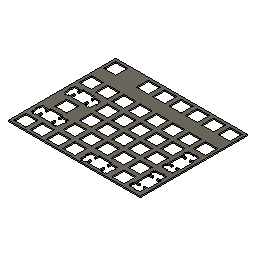
keeb plate v2 (Autodesk Fusion 360 design; units mm, degrees)
Autodesk Fusion 360 part; units mm, degrees
sketch "Sketch1" plane through (0, 0, 0) normal (0, 0, 1) x (1, 0, 0)
  line L0 (93.2552, -112.3061) -> (93.2552, -117.0063)
  line L1 (93.2552, -117.0063) -> (91.7301, -117.0063)
  line L2 (91.7301, -117.0063) -> (91.7301, -113.7761)
  line L3 (91.7301, -113.7761) -> (84.9798, -113.7761)
  line L4 (84.9798, -113.7761) -> (84.9798, -117.0063)
  line L5 (84.9798, -117.0063) -> (84.1548, -117.0063)
  line L6 (84.1548, -117.0063) -> (84.1548, -119.8064)
  line L7 (84.1548, -119.8064) -> (84.9798, -119.8064)
  line L8 (84.9798, -119.8064) -> (84.9798, -126.0767)
  line L9 (84.9798, -126.0767) -> (86.7049, -126.0767)
  line L10 (86.7049, -126.0767) -> (86.7049, -127.2767)
  line L11 (86.7049, -127.2767) -> (90.005, -127.2767)
  line L12 (90.005, -127.2767) -> (90.005, -126.0767)
  line L13 (90.005, -126.0767) -> (91.7301, -126.0767)
  line L14 (91.7301, -126.0767) -> (91.7301, -121.6065)
  line L15 (91.7301, -121.6065) -> (93.2552, -121.6065)
  line L16 (93.2552, -121.6065) -> (93.2552, -126.3067)
  line L17 (93.2552, -126.3067) -> (107.2558, -126.3067)
  line L18 (107.2558, -126.3067) -> (107.2558, -121.6065)
  line L19 (107.2558, -121.6065) -> (108.7809, -121.6065)
  line L20 (108.7809, -121.6065) -> (108.7809, -126.0767)
  line L21 (108.7809, -126.0767) -> (110.506, -126.0767)
  line L22 (110.506, -126.0767) -> (110.506, -127.2767)
  line L23 (110.506, -127.2767) -> (113.8061, -127.2767)
  line L24 (113.8061, -127.2767) -> (113.8061, -126.0767)
  line L25 (113.8061, -126.0767) -> (115.5312, -126.0767)
  line L26 (115.5312, -126.0767) -> (115.5312, -119.8064)
  line L27 (115.5312, -119.8064) -> (116.3562, -119.8064)
  line L28 (116.3562, -119.8064) -> (116.3562, -117.0063)
  line L29 (116.3562, -117.0063) -> (115.5312, -117.0063)
  line L30 (115.5312, -117.0063) -> (115.5312, -113.7761)
  line L31 (115.5312, -113.7761) -> (108.7809, -113.7761)
  line L32 (108.7809, -113.7761) -> (108.7809, -117.0063)
  line L33 (108.7809, -117.0063) -> (107.2558, -117.0063)
  line L34 (107.2558, -117.0063) -> (107.2558, -112.3061)
  line L35 (107.2558, -112.3061) -> (93.2552, -112.3061)
  line L36 (121.8305, -112.3061) -> (121.8305, -126.3067)
  line L37 (121.8305, -126.3067) -> (135.8321, -126.3067)
  line L38 (135.8321, -126.3067) -> (135.8321, -112.3061)
  line L39 (135.8321, -112.3061) -> (121.8305, -112.3061)
  line L40 (64.6789, -112.3061) -> (64.6789, -126.3067)
  line L41 (64.6789, -126.3067) -> (78.6795, -126.3067)
  line L42 (78.6795, -126.3067) -> (78.6795, -112.3061)
  line L43 (78.6795, -112.3061) -> (64.6789, -112.3061)
  line L44 (45.6281, -112.3061) -> (45.6281, -126.3067)
  line L45 (45.6281, -126.3067) -> (59.6287, -126.3067)
  line L46 (59.6287, -126.3067) -> (59.6287, -112.3061)
  line L47 (59.6287, -112.3061) -> (45.6281, -112.3061)
  line L48 (26.5772, -112.3061) -> (26.5772, -126.3067)
  line L49 (26.5772, -126.3067) -> (40.5778, -126.3067)
  line L50 (40.5778, -126.3067) -> (40.5778, -112.3061)
  line L51 (40.5778, -112.3061) -> (26.5772, -112.3061)
  line L52 (7.5263, -112.3061) -> (7.5263, -126.3067)
  line L53 (7.5263, -126.3067) -> (21.527, -126.3067)
  line L54 (21.527, -126.3067) -> (21.527, -112.3061)
  line L55 (21.527, -112.3061) -> (7.5263, -112.3061)
  line L56 (147.3826, -93.6802) -> (147.3826, -94.5053)
  line L57 (147.3826, -94.5053) -> (141.1123, -94.5053)
  line L58 (141.1123, -94.5053) -> (141.1123, -96.2303)
  line L59 (141.1123, -96.2303) -> (139.9123, -96.2303)
  line L60 (139.9123, -96.2303) -> (139.9123, -99.5305)
  line L61 (139.9123, -99.5305) -> (141.1123, -99.5305)
  line L62 (141.1123, -99.5305) -> (141.1123, -101.2556)
  line L63 (141.1123, -101.2556) -> (145.5826, -101.2556)
  line L64 (145.5826, -101.2556) -> (145.5826, -102.7806)
  line L65 (145.5826, -102.7806) -> (140.8823, -102.7806)
  line L66 (140.8823, -102.7806) -> (140.8823, -116.7813)
  line L67 (140.8823, -116.7813) -> (145.5826, -116.7813)
  line L68 (145.5826, -116.7813) -> (145.5826, -118.3063)
  line L69 (145.5826, -118.3063) -> (141.1123, -118.3063)
  line L70 (141.1123, -118.3063) -> (141.1123, -120.0314)
  line L71 (141.1123, -120.0314) -> (139.9123, -120.0314)
  line L72 (139.9123, -120.0314) -> (139.9123, -123.3315)
  line L73 (139.9123, -123.3315) -> (141.1123, -123.3315)
  line L74 (141.1123, -123.3315) -> (141.1123, -125.0566)
  line L75 (141.1123, -125.0566) -> (147.3826, -125.0566)
  line L76 (147.3826, -125.0566) -> (147.3826, -125.8817)
  line L77 (147.3826, -125.8817) -> (150.1828, -125.8817)
  line L78 (150.1828, -125.8817) -> (150.1828, -125.0566)
  line L79 (150.1828, -125.0566) -> (153.4129, -125.0566)
  line L80 (153.4129, -125.0566) -> (153.4129, -118.3063)
  line L81 (153.4129, -118.3063) -> (150.1828, -118.3063)
  line L82 (150.1828, -118.3063) -> (150.1828, -116.7813)
  line L83 (150.1828, -116.7813) -> (154.883, -116.7813)
  line L84 (154.883, -116.7813) -> (154.883, -102.7806)
  line L85 (154.883, -102.7806) -> (150.1828, -102.7806)
  line L86 (150.1828, -102.7806) -> (150.1828, -101.2556)
  line L87 (150.1828, -101.2556) -> (153.4129, -101.2556)
  line L88 (153.4129, -101.2556) -> (153.4129, -94.5053)
  line L89 (153.4129, -94.5053) -> (150.1828, -94.5053)
  line L90 (150.1828, -94.5053) -> (150.1828, -93.6802)
  line L91 (150.1828, -93.6802) -> (147.3826, -93.6802)
  line L92 (17.0518, -93.2552) -> (17.0518, -97.9554)
  line L93 (17.0518, -97.9554) -> (15.5267, -97.9554)
  line L94 (15.5267, -97.9554) -> (15.5267, -94.7253)
  line L95 (15.5267, -94.7253) -> (8.7764, -94.7253)
  line L96 (8.7764, -94.7253) -> (8.7764, -97.9554)
  line L97 (8.7764, -97.9554) -> (7.9504, -97.9554)
  line L98 (7.9504, -97.9554) -> (7.9504, -100.7555)
  line L99 (7.9504, -100.7555) -> (8.7764, -100.7555)
  line L100 (8.7764, -100.7555) -> (8.7764, -107.0258)
  line L101 (8.7764, -107.0258) -> (10.5015, -107.0258)
  line L102 (10.5015, -107.0258) -> (10.5015, -108.2259)
  line L103 (10.5015, -108.2259) -> (13.8016, -108.2259)
  line L104 (13.8016, -108.2259) -> (13.8016, -107.0258)
  line L105 (13.8016, -107.0258) -> (15.5267, -107.0258)
  line L106 (15.5267, -107.0258) -> (15.5267, -102.5556)
  line L107 (15.5267, -102.5556) -> (17.0518, -102.5556)
  line L108 (17.0518, -102.5556) -> (17.0518, -107.2558)
  line L109 (17.0518, -107.2558) -> (31.0524, -107.2558)
  line L110 (31.0524, -107.2558) -> (31.0524, -102.5556)
  line L111 (31.0524, -102.5556) -> (32.5775, -102.5556)
  line L112 (32.5775, -102.5556) -> (32.5775, -107.0258)
  line L113 (32.5775, -107.0258) -> (34.3025, -107.0258)
  line L114 (34.3025, -107.0258) -> (34.3025, -108.2259)
  line L115 (34.3025, -108.2259) -> (37.6027, -108.2259)
  line L116 (37.6027, -108.2259) -> (37.6027, -107.0258)
  line L117 (37.6027, -107.0258) -> (39.3278, -107.0258)
  line L118 (39.3278, -107.0258) -> (39.3278, -100.7555)
  line L119 (39.3278, -100.7555) -> (40.1528, -100.7555)
  line L120 (40.1528, -100.7555) -> (40.1528, -97.9554)
  line L121 (40.1528, -97.9554) -> (39.3278, -97.9554)
  line L122 (39.3278, -97.9554) -> (39.3278, -94.7253)
  line L123 (39.3278, -94.7253) -> (32.5775, -94.7253)
  line L124 (32.5775, -94.7253) -> (32.5775, -97.9554)
  line L125 (32.5775, -97.9554) -> (31.0524, -97.9554)
  line L126 (31.0524, -97.9554) -> (31.0524, -93.2552)
  line L127 (31.0524, -93.2552) -> (17.0518, -93.2552)
  line L128 (121.8305, -93.2552) -> (121.8305, -107.2558)
  line L129 (121.8305, -107.2558) -> (135.8321, -107.2558)
  line L130 (135.8321, -107.2558) -> (135.8321, -93.2552)
  line L131 (135.8321, -93.2552) -> (121.8305, -93.2552)
  line L132 (102.7796, -93.2552) -> (102.7796, -107.2558)
  line L133 (102.7796, -107.2558) -> (116.7803, -107.2558)
  line L134 (116.7803, -107.2558) -> (116.7803, -93.2552)
  line L135 (116.7803, -93.2552) -> (102.7796, -93.2552)
  line L136 (83.7298, -93.2552) -> (83.7298, -107.2558)
  line L137 (83.7298, -107.2558) -> (97.7304, -107.2558)
  line L138 (97.7304, -107.2558) -> (97.7304, -93.2552)
  line L139 (97.7304, -93.2552) -> (83.7298, -93.2552)
  line L140 (64.6789, -93.2552) -> (64.6789, -107.2558)
  line L141 (64.6789, -107.2558) -> (78.6795, -107.2558)
  line L142 (78.6795, -107.2558) -> (78.6795, -93.2552)
  line L143 (78.6795, -93.2552) -> (64.6789, -93.2552)
  line L144 (45.6281, -93.2552) -> (45.6281, -107.2558)
  line L145 (45.6281, -107.2558) -> (59.6287, -107.2558)
  line L146 (59.6287, -107.2558) -> (59.6287, -93.2552)
  line L147 (59.6287, -93.2552) -> (45.6281, -93.2552)
  line L148 (121.8305, -74.2043) -> (121.8305, -88.205)
  line L149 (121.8305, -88.205) -> (135.8321, -88.205)
  line L150 (135.8321, -88.205) -> (135.8321, -74.2043)
  line L151 (135.8321, -74.2043) -> (121.8305, -74.2043)
  line L152 (102.7796, -74.2043) -> (102.7796, -88.205)
  line L153 (102.7796, -88.205) -> (116.7803, -88.205)
  line L154 (116.7803, -88.205) -> (116.7803, -74.2043)
  line L155 (116.7803, -74.2043) -> (102.7796, -74.2043)
  line L156 (83.7298, -74.2043) -> (83.7298, -88.205)
  line L157 (83.7298, -88.205) -> (97.7304, -88.205)
  line L158 (97.7304, -88.205) -> (97.7304, -74.2043)
  line L159 (97.7304, -74.2043) -> (83.7298, -74.2043)
  line L160 (64.6789, -74.2043) -> (64.6789, -88.205)
  line L161 (64.6789, -88.205) -> (78.6795, -88.205)
  line L162 (78.6795, -88.205) -> (78.6795, -74.2043)
  line L163 (78.6795, -74.2043) -> (64.6789, -74.2043)
  line L164 (45.6281, -74.2043) -> (45.6281, -88.205)
  line L165 (45.6281, -88.205) -> (59.6287, -88.205)
  line L166 (59.6287, -88.205) -> (59.6287, -74.2043)
  line L167 (59.6287, -74.2043) -> (45.6281, -74.2043)
  line L168 (17.0508, -74.2043) -> (17.0508, -88.205)
  line L169 (17.0508, -88.205) -> (31.0514, -88.205)
  line L170 (31.0514, -88.205) -> (31.0514, -74.2043)
  line L171 (31.0514, -74.2043) -> (17.0508, -74.2043)
  line L172 (147.3826, -55.5785) -> (147.3826, -56.4035)
  line L173 (147.3826, -56.4035) -> (141.1123, -56.4035)
  line L174 (141.1123, -56.4035) -> (141.1123, -58.1286)
  line L175 (141.1123, -58.1286) -> (139.9123, -58.1286)
  line L176 (139.9123, -58.1286) -> (139.9123, -61.4288)
  line L177 (139.9123, -61.4288) -> (141.1123, -61.4288)
  line L178 (141.1123, -61.4288) -> (141.1123, -63.1538)
  line L179 (141.1123, -63.1538) -> (145.5826, -63.1538)
  line L180 (145.5826, -63.1538) -> (145.5826, -64.6789)
  line L181 (145.5826, -64.6789) -> (140.8823, -64.6789)
  line L182 (140.8823, -64.6789) -> (140.8823, -78.6795)
  line L183 (140.8823, -78.6795) -> (145.5826, -78.6795)
  line L184 (145.5826, -78.6795) -> (145.5826, -80.2046)
  line L185 (145.5826, -80.2046) -> (141.1123, -80.2046)
  line L186 (141.1123, -80.2046) -> (141.1123, -81.9297)
  line L187 (141.1123, -81.9297) -> (139.9123, -81.9297)
  line L188 (139.9123, -81.9297) -> (139.9123, -85.2298)
  line L189 (139.9123, -85.2298) -> (141.1123, -85.2298)
  line L190 (141.1123, -85.2298) -> (141.1123, -86.9549)
  line L191 (141.1123, -86.9549) -> (147.3826, -86.9549)
  line L192 (147.3826, -86.9549) -> (147.3826, -87.7799)
  line L193 (147.3826, -87.7799) -> (150.1828, -87.7799)
  line L194 (150.1828, -87.7799) -> (150.1828, -86.9549)
  line L195 (150.1828, -86.9549) -> (153.4129, -86.9549)
  line L196 (153.4129, -86.9549) -> (153.4129, -80.2046)
  line L197 (153.4129, -80.2046) -> (150.1828, -80.2046)
  line L198 (150.1828, -80.2046) -> (150.1828, -78.6795)
  line L199 (150.1828, -78.6795) -> (154.883, -78.6795)
  line L200 (154.883, -78.6795) -> (154.883, -64.6789)
  line L201 (154.883, -64.6789) -> (150.1828, -64.6789)
  line L202 (150.1828, -64.6789) -> (150.1828, -63.1538)
  line L203 (150.1828, -63.1538) -> (153.4129, -63.1538)
  line L204 (153.4129, -63.1538) -> (153.4129, -56.4035)
  line L205 (153.4129, -56.4035) -> (150.1828, -56.4035)
  line L206 (150.1828, -56.4035) -> (150.1828, -55.5785)
  line L207 (150.1828, -55.5785) -> (147.3826, -55.5785)
  line L208 (17.0518, -55.1535) -> (17.0518, -59.8537)
  line L209 (17.0518, -59.8537) -> (15.5267, -59.8537)
  line L210 (15.5267, -59.8537) -> (15.5267, -56.6235)
  line L211 (15.5267, -56.6235) -> (8.7764, -56.6235)
  line L212 (8.7764, -56.6235) -> (8.7764, -59.8537)
  line L213 (8.7764, -59.8537) -> (7.9504, -59.8537)
  line L214 (7.9504, -59.8537) -> (7.9504, -62.6538)
  line L215 (7.9504, -62.6538) -> (8.7764, -62.6538)
  line L216 (8.7764, -62.6538) -> (8.7764, -68.9241)
  line L217 (8.7764, -68.9241) -> (10.5015, -68.9241)
  line L218 (10.5015, -68.9241) -> (10.5015, -70.1242)
  line L219 (10.5015, -70.1242) -> (13.8016, -70.1242)
  line L220 (13.8016, -70.1242) -> (13.8016, -68.9241)
  line L221 (13.8016, -68.9241) -> (15.5267, -68.9241)
  line L222 (15.5267, -68.9241) -> (15.5267, -64.4539)
  line L223 (15.5267, -64.4539) -> (17.0518, -64.4539)
  line L224 (17.0518, -64.4539) -> (17.0518, -69.1541)
  line L225 (17.0518, -69.1541) -> (31.0524, -69.1541)
  line L226 (31.0524, -69.1541) -> (31.0524, -64.4539)
  line L227 (31.0524, -64.4539) -> (32.5775, -64.4539)
  line L228 (32.5775, -64.4539) -> (32.5775, -68.9241)
  line L229 (32.5775, -68.9241) -> (34.3025, -68.9241)
  line L230 (34.3025, -68.9241) -> (34.3025, -70.1242)
  line L231 (34.3025, -70.1242) -> (37.6027, -70.1242)
  line L232 (37.6027, -70.1242) -> (37.6027, -68.9241)
  line L233 (37.6027, -68.9241) -> (39.3278, -68.9241)
  line L234 (39.3278, -68.9241) -> (39.3278, -62.6538)
  line L235 (39.3278, -62.6538) -> (40.1528, -62.6538)
  line L236 (40.1528, -62.6538) -> (40.1528, -59.8537)
  line L237 (40.1528, -59.8537) -> (39.3278, -59.8537)
  line L238 (39.3278, -59.8537) -> (39.3278, -56.6235)
  line L239 (39.3278, -56.6235) -> (32.5775, -56.6235)
  line L240 (32.5775, -56.6235) -> (32.5775, -59.8537)
  line L241 (32.5775, -59.8537) -> (31.0524, -59.8537)
  line L242 (31.0524, -59.8537) -> (31.0524, -55.1535)
  line L243 (31.0524, -55.1535) -> (17.0518, -55.1535)
  line L244 (121.8305, -55.1535) -> (121.8305, -69.1541)
  line L245 (121.8305, -69.1541) -> (135.8321, -69.1541)
  line L246 (135.8321, -69.1541) -> (135.8321, -55.1535)
  line L247 (135.8321, -55.1535) -> (121.8305, -55.1535)
  line L248 (102.7796, -55.1535) -> (102.7796, -69.1541)
  line L249 (102.7796, -69.1541) -> (116.7803, -69.1541)
  line L250 (116.7803, -69.1541) -> (116.7803, -55.1535)
  line L251 (116.7803, -55.1535) -> (102.7796, -55.1535)
  line L252 (83.7298, -55.1535) -> (83.7298, -69.1541)
  line L253 (83.7298, -69.1541) -> (97.7304, -69.1541)
  line L254 (97.7304, -69.1541) -> (97.7304, -55.1535)
  line L255 (97.7304, -55.1535) -> (83.7298, -55.1535)
  line L256 (64.6789, -55.1535) -> (64.6789, -69.1541)
  line L257 (64.6789, -69.1541) -> (78.6795, -69.1541)
  line L258 (78.6795, -69.1541) -> (78.6795, -55.1535)
  line L259 (78.6795, -55.1535) -> (64.6789, -55.1535)
  line L260 (45.6281, -55.1535) -> (45.6281, -69.1541)
  line L261 (45.6281, -69.1541) -> (59.6287, -69.1541)
  line L262 (59.6287, -69.1541) -> (59.6287, -55.1535)
  line L263 (59.6287, -55.1535) -> (45.6281, -55.1535)
  line L264 (140.8823, -36.1026) -> (140.8823, -50.1033)
  line L265 (140.8823, -50.1033) -> (154.883, -50.1033)
  line L266 (154.883, -50.1033) -> (154.883, -36.1026)
  line L267 (154.883, -36.1026) -> (140.8823, -36.1026)
  line L268 (121.8305, -36.1026) -> (121.8305, -50.1033)
  line L269 (121.8305, -50.1033) -> (135.8321, -50.1033)
  line L270 (135.8321, -50.1033) -> (135.8321, -36.1026)
  line L271 (135.8321, -36.1026) -> (121.8305, -36.1026)
  line L272 (102.7796, -36.1026) -> (102.7796, -50.1033)
  line L273 (102.7796, -50.1033) -> (116.7803, -50.1033)
  line L274 (116.7803, -50.1033) -> (116.7803, -36.1026)
  line L275 (116.7803, -36.1026) -> (102.7796, -36.1026)
  line L276 (83.7298, -36.1026) -> (83.7298, -50.1033)
  line L277 (83.7298, -50.1033) -> (97.7304, -50.1033)
  line L278 (97.7304, -50.1033) -> (97.7304, -36.1026)
  line L279 (97.7304, -36.1026) -> (83.7298, -36.1026)
  line L280 (64.6789, -36.1026) -> (64.6789, -50.1033)
  line L281 (64.6789, -50.1033) -> (78.6795, -50.1033)
  line L282 (78.6795, -50.1033) -> (78.6795, -36.1026)
  line L283 (78.6795, -36.1026) -> (64.6789, -36.1026)
  line L284 (45.6281, -36.1026) -> (45.6281, -50.1033)
  line L285 (45.6281, -50.1033) -> (59.6287, -50.1033)
  line L286 (59.6287, -50.1033) -> (59.6287, -36.1026)
  line L287 (59.6287, -36.1026) -> (45.6281, -36.1026)
  line L288 (26.5772, -36.1026) -> (26.5772, -50.1033)
  line L289 (26.5772, -50.1033) -> (40.5778, -50.1033)
  line L290 (40.5778, -50.1033) -> (40.5778, -36.1026)
  line L291 (40.5778, -36.1026) -> (26.5772, -36.1026)
  line L292 (7.5263, -36.1026) -> (7.5263, -50.1033)
  line L293 (7.5263, -50.1033) -> (21.527, -50.1033)
  line L294 (21.527, -50.1033) -> (21.527, -36.1026)
  line L295 (21.527, -36.1026) -> (7.5263, -36.1026)
  line L296 (140.8823, -7.5263) -> (140.8823, -21.527)
  line L297 (140.8823, -21.527) -> (154.883, -21.527)
  line L298 (154.883, -21.527) -> (154.883, -7.5263)
  line L299 (154.883, -7.5263) -> (140.8823, -7.5263)
  line L300 (121.8305, -7.5263) -> (121.8305, -21.527)
  line L301 (121.8305, -21.527) -> (135.8321, -21.527)
  line L302 (135.8321, -21.527) -> (135.8321, -7.5263)
  line L303 (135.8321, -7.5263) -> (121.8305, -7.5263)
  line L304 (102.7796, -7.5263) -> (102.7796, -21.527)
  line L305 (102.7796, -21.527) -> (116.7803, -21.527)
  line L306 (116.7803, -21.527) -> (116.7803, -7.5263)
  line L307 (116.7803, -7.5263) -> (102.7796, -7.5263)
  line L308 (83.7298, -7.5263) -> (83.7298, -21.527)
  line L309 (83.7298, -21.527) -> (97.7304, -21.527)
  line L310 (97.7304, -21.527) -> (97.7304, -7.5263)
  line L311 (97.7304, -7.5263) -> (83.7298, -7.5263)
  line L312 (64.6789, -7.5263) -> (64.6789, -21.527)
  line L313 (64.6789, -21.527) -> (78.6795, -21.527)
  line L314 (78.6795, -21.527) -> (78.6795, -7.5263)
  line L315 (78.6795, -7.5263) -> (64.6789, -7.5263)
  line L316 (45.6281, -7.5263) -> (45.6281, -21.527)
  line L317 (45.6281, -21.527) -> (59.6287, -21.527)
  line L318 (59.6287, -21.527) -> (59.6287, -7.5263)
  line L319 (59.6287, -7.5263) -> (45.6281, -7.5263)
  line L320 (7.5263, -7.5263) -> (7.5263, -21.527)
  line L321 (7.5263, -21.527) -> (21.527, -21.527)
  line L322 (21.527, -21.527) -> (21.527, -7.5263)
  line L323 (21.527, -7.5263) -> (7.5263, -7.5263)
  line L324 (4.3552, -20.6751) -> (4.3362, -4.3714)
  line L325 (11.8957, -4.3589) -> (4.3362, -4.3678)
  line L326 (4.3362, -4.3678) -> (4.3362, -4.3714)
  line L327 (15.0751, -4.3568) -> (158.053, -4.3568)
  line L328 (158.053, -4.3568) -> (158.053, -14.5267)
  line L329 (4.3552, -20.6751) -> (4.3561, -129.4767)
  line L330 (87.604, -129.4761) -> (4.3561, -129.4767)
  line L331 (87.604, -129.4761) -> (158.0745, -129.4761)
  line L332 (158.053, -109.7809) -> (158.053, -129.4761)
  line L333 (158.053, -109.7809) -> (158.053, -14.5267)
  line L334 (11.8957, -4.3589) -> (15.0751, -4.3568)
  constraint perpendicular L325 L326
  constraint perpendicular L316 L327
  constraint coincident L327 L328.start
  constraint coincident L329 L330.end
  constraint perpendicular L329 L330
  constraint coincident L331 L332.end
  constraint perpendicular L331 L332
  constraint perpendicular L327 L328
extrude "Extrude1" add sketch "Sketch1" along normal blind 1.5
sketch "Sketch2" plane through (0, 0, 0) normal (0, 0, 1) x (1, 0, 0)
